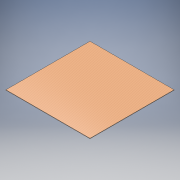
# Autodesk Inventor part: floor_50_100
Saved by Autodesk Inventor 2019 (Build 230136000, 136)
## iProperties
Created: 2020-04-28
Part Number: floor_50_100
Material: Wood (Birch)
Document SubType Name: Modeling
Designer: infinity
Density: 0.55 g/cm^3
Appearance: Birch - Natural Polished
Author: infinity
Autodesk Inventor part; units mm, degrees
ref_plane "YZ Plane" through (0, 0, 0) normal (1, 0, 0) x (0, 1, 0)
ref_plane "XZ Plane" through (0, 0, 0) normal (0, 1, 0) x (-1, 0, 0)
ref_plane "XY Plane" through (0, 0, 0) normal (0, 0, 1) x (1, 0, 0)
sketch "Sketch1" plane through (0, 0, 0) normal (0, 1, 0) x (-1, 0, 0)
  line L0 (0, 0) -> (15240, 0)
  line L1 (15240, 0) -> (15240, -15240)
  line L2 (15240, -15240) -> (0, -15240)
  line L3 (0, -15240) -> (0, 0)
  dimension "d0" = 15240
  dimension "d1" = 15240
  constraints: 8 end point, 2 parallel, 1 horizontal, 1 perpendicular
  measures "d0" distance of L0.end L1.end
  measures "d1" distance of L0.start L0.end
extrude "Extrusion1" add sketch "Sketch1" along normal blind 76.2
body "Solid1"
